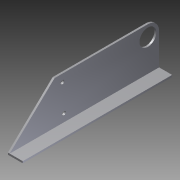
# Autodesk Inventor part: apendage L bracket left
Saved by Autodesk Inventor 2012 (Build 160160000, 160)
## iProperties
Created: 2013-07-07
Part Number: apendage L bracket left
Material: Default
Document SubType Name: Modeling
Designer: Bryce
Density: 1 g/cm^3
Author: Bryce
Autodesk Inventor part; units mm, degrees
ref_plane "YZ Plane" through (0, 0, 0) normal (1, 0, 0) x (0, 1, 0)
ref_plane "XZ Plane" through (0, 0, 0) normal (0, 1, 0) x (-1, 0, 0)
ref_plane "XY Plane" through (0, 0, 0) normal (0, 0, 1) x (1, 0, 0)
sketch "Sketch1" plane through (0, 0, 0) normal (0, 0, 1) x (1, 0, 0)
  line L0 (0, 0) -> (25.4, 0)
  line L1 (0, 76.2) -> (0, 0)
  line L2 (25.4, 3.175) -> (3.175, 3.175)
  line L3 (3.175, 3.175) -> (3.175, 76.2)
  line L4 (0, 76.2) -> (3.175, 76.2)
  line L5 (25.4, 3.175) -> (25.4, 0)
  dimension "d0" = 76.2
  dimension "d1" = 25.4
  dimension "d2" = 3.175
  dimension "d3" = 3.175
  constraints: 12 end point, 3 perpendicular, 1 horizontal
  measures "d0" distance of L1.start L0.start
  measures "d1" distance of L0.start L0.end
  measures "d2" distance between parallel lines of L1 L3
  measures "d3" distance between parallel lines of L0 L2
extrude "Extrusion1" add sketch "Sketch1" along normal blind 254
sketch "Sketch2" plane through (3.175, 3.175, 0) normal (1, 0, 0) x (0, 0, -1)
  line L0 (-254, 73.025) -> (-254, 0) projected
  line L1 (0, 73.025) -> (-254, 73.025) projected
  line L2 (0, 0) -> (-254, 0) projected
  line L3 (0, -3.175) -> (-254, -3.175) projected
  line L4 (-254, 0) -> (-254, -3.175) projected
  line L5 (0, -3.175) -> (0, 0) projected
  line L6 (-254, 0) -> (-177.8, 73.025)
  line L7 (-177.8, 73.025) -> (-173.7896, 0) construction
  line L8 (-152.3617, 73.025) -> (-148.4278, 1.3928) construction
  line L9 (-148.4278, 1.3928) -> (-173.7896, 0) construction
  circle A0 centre (-161.8051, 13.3773) radius 3.175
  circle A1 centre (-164.3834, 60.325) radius 3.175
  line L10 (0, 0) -> (0, 73.025) projected
  arc A2 (0, 53.975) -> (-19.05, 73.025) centre (-19.05, 53.975) ccw
  circle A3 centre (-19.05, 53.975) radius 14.2875
  dimension "d6" = 25.4
  dimension "d7" = 12.7
  dimension "d8" = 76.2
  dimension "d9" = 12.7
  dimension "d10" = 12.7
  dimension "d11" = 12.7
  dimension "d12" = 12.7
  dimension "d13" = 6.35
  dimension "d14" = 6.35
  dimension "d17" = 19.05
  dimension "d18" = 28.575
  dimension "d19" = 3.143
  constraints: 8 end point, 5 point on line, 4 centre point, 2 coincident, 2 point on circle, 2 tangent, 1 parallel, 1 perpendicular
  measures "d6" distance between parallel lines of L8 L7
  measures "d7" distance from line of L9 point (0, -3.175)
  measures "d8" distance from line of L0 L6.end
  measures "d9" distance from line of L1 A1.centre
  measures "d10" distance from line of L9 A0.centre
  measures "d11" distance from line of L7 A1.centre
  measures "d12" distance from line of L7 A0.centre
  measures "d13" diameter of A1
  measures "d14" diameter of A0
  measures "d17" radius of A2
  measures "d18" diameter of A3
  measures "d19" angle of L2 L9
extrude "Extrusion2" cut sketch "Sketch2" against normal blind 25.4 contours L1 L6 L0 | L1 L10 A2 | A0 | A1 | A3
equation "\"d3\" = d2"
equation "\"d10\" = d9"
equation "\"d11\" = 0.5 * d6"
equation "\"d12\" = d11"
equation "\"d14\" = d13"
body "Solid1"
